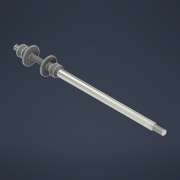
# Autodesk Inventor part: tłoczysko
Saved by Autodesk Inventor 2022 (Build 260153000, 153)
## iProperties
Created: 2023-04-12
Part Number: tłoczysko
Material: Ogólny
Document SubType Name: Modeling
Designer: jacek
Density: 1 g/cm^3
Appearance: Gładki — czarny
Author: jacek
Autodesk Inventor part; units mm, degrees
ref_plane "YZ Plane" through (0, 0, 0) normal (1, 0, 0) x (0, 1, 0)
ref_plane "XY Plane" through (0, 0, 0) normal (0, 0, 1) x (1, 0, 0)
sketch "Szkic1" plane through (0, 0, 0) normal (1, 0, 0) x (0, 1, 0)
  circle A0 centre (0, 0) radius 7
  dimension "d0" = 14
  constraints: 1 centre point, 1 coincident
  measures "d0" diameter of A0
extrude "Wyciągnięcie proste1" add sketch "Szkic1" along normal blind 100
sketch "Szkic2" plane through (100, 0, 0) normal (1, 0, 0) x (0, 0, -1)
  circle A0 centre (0, 0) radius 25.5
  dimension "d3" = 51
  constraints: 1 centre point, 1 coincident
  measures "d3" diameter of A0
extrude "Wyciągnięcie proste2" add sketch "Szkic2" against normal blind 3
ref_plane "Płaszczyzna konstrukcyjna1" through (43, 0, 0) normal (-1, 0, 0) x (0, 0, 1)
sketch "Szkic3" plane through (43, 0, 0) normal (-1, 0, 0) x (0, 0, 1)
  circle A0 centre (0, 0) radius 25.5
  constraints: 1 centre point, 1 coincident
extrude "Wyciągnięcie proste3" add sketch "Szkic3" along normal blind 3
sketch "Szkic4" plane through (40, 0, 0) normal (-1, 0, 0) x (0, 0, 1)
  circle A0 centre (0, 0) radius 10
  dimension "d9" = 20
  constraints: 1 centre point, 1 coincident
  measures "d9" diameter of A0
extrude "Wyciągnięcie proste4" add sketch "Szkic4" along normal blind 9
sketch "Szkic5" plane through (31, 0, 0) normal (-1, 0, 0) x (0, 0, 1)
  circle A0 centre (0, 0) radius 13.5
  dimension "d12" = 27
  constraints: 1 centre point, 1 coincident
  measures "d12" diameter of A0
extrude "Wyciągnięcie proste5" add sketch "Szkic5" along normal blind 11
fillet "Zaokrąglenie1" radius 8 1 edges at (31, 0, -13.5)
ref_plane "Płaszczyzna konstrukcyjna2" through (10, 0, 0) normal (-1, 0, 0) x (0, 0, 1)
sketch "Szkic6" plane through (10, 0, 0) normal (-1, 0, 0) x (0, 0, 1)
  circle A0 centre (0, 0) radius 14.5
  dimension "d19" = 29
  constraints: 1 centre point, 1 coincident
  measures "d19" diameter of A0
extrude "Wyciągnięcie proste6" add sketch "Szkic6" against normal blind 1
sketch "Szkic7" plane through (11, 0, 0) normal (1, 0, 0) x (0, 0, -1)
  circle A0 centre (0, 0) radius 15
  dimension "d22" = 30
  constraints: 1 centre point, 1 coincident
  measures "d22" diameter of A0
extrude "Wyciągnięcie proste7" add sketch "Szkic7" along normal blind 1
sketch "Szkic8" plane through (12, 0, 0) normal (1, 0, 0) x (0, 0, -1)
  circle A0 centre (0, 0) radius 7 projected
  circle A1 centre (0, 0) radius 15.75
  circle A2 centre (0, 0) radius 13.5 projected
  circle A3 centre (0, 0) radius 14.5
  dimension "d25" = 31.5
  constraints: 2 centre point, 2 coincident
  measures "d25" diameter of A1
extrude "Wyciągnięcie proste8" add sketch "Szkic8" along normal blind 13 contours A1
extrude "Wyciągnięcie proste9" add sketch "Szkic8" along normal blind 7.75 contours A0 | A2 | A3
sketch "Szkic9" plane through (100, 0, 0) normal (1, 0, 0) x (0, 0, -1)
  circle A0 centre (0, 0) radius 7
  circle A1 centre (0, 0) radius 10
  dimension "d30" = 14
  dimension "d33" = 20
  constraints: 2 centre point, 2 coincident
  measures "d30" diameter of A0
  measures "d33" diameter of A1
extrude "Wyciągnięcie proste10" add sketch "Szkic9" along normal blind 23 contours A0
extrude "Wyciągnięcie proste11" add sketch "Szkic9" along normal blind 9
sketch "Szkic10" plane through (109, 0, 0) normal (1, 0, 0) x (0, 0, -1)
  circle A0 centre (0, 0) radius 25.5 projected
  circle A1 centre (0, 0) radius 13.5
  dimension "d36" = 27
  constraints: 1 centre point, 1 coincident
  measures "d36" diameter of A1
extrude "Wyciągnięcie proste12" add sketch "Szkic10" along normal blind 11 contours A1
fillet "Zaokrąglenie2" radius 8 1 edges at (109, 0, 13.5)
ref_plane "Płaszczyzna konstrukcyjna3" through (115.5, 0, 0) normal (1, 0, 0) x (0, 0, -1)
sketch "Szkic11" plane through (115.5, 0, 0) normal (1, 0, 0) x (0, 0, -1)
  circle A0 centre (0, 0) radius 15.75
  circle A1 centre (0, 0) radius 14.5
  dimension "d41" = 31.5
  dimension "d42" = 29
  constraints: 2 centre point, 2 coincident
  measures "d41" diameter of A0
  measures "d42" diameter of A1
extrude "Wyciągnięcie proste13" add sketch "Szkic11" along normal blind 13
sketch "Szkic12" plane through (123, 0, 0) normal (1, 0, 0) x (0, 0, -1)
  circle A0 centre (0, 0) radius 10
  dimension "d45" = 20
  constraints: 1 centre point, 1 coincident
  measures "d45" diameter of A0
extrude "Wyciągnięcie proste14" add sketch "Szkic12" along normal blind 350
ref_plane "Płaszczyzna konstrukcyjna4" through (128.5, 0, 0) normal (1, 0, 0) x (0, 0, -1)
sketch "Szkic13" plane through (128.5, 0, 0) normal (1, 0, 0) x (0, 0, -1)
  circle A0 centre (0, 0) radius 15.75
  constraints: 1 centre point, 1 coincident
extrude "Wyciągnięcie proste15" add sketch "Szkic13" along normal blind 8
fillet "Zaokrąglenie3" radius 8 1 edges at (136.5, 0, 15.75)
sketch "Szkic14" plane through (473, 0, 0) normal (1, 0, 0) x (0, 0, -1)
  circle A0 centre (0, 0) radius 7.5
  circle A1 centre (0, 0) radius 18.8953
  dimension "d52" = 15
  constraints: 2 centre point, 2 coincident
  measures "d52" diameter of A0
extrude "Wyciągnięcie proste16" cut sketch "Szkic14" against normal blind 35
thread "Gwint2" size "M15x1.5" class "6g" standard "ANSI Metric M Profile" length 33
chamfer "Faza1" distance 2 angle 45 2 edges at (473, 0, 7.5) (438, 0, 10)
ref_plane "Płaszczyzna konstrukcyjna5" through (123, 10, 0) normal (0, 1, 0) x (-1, 0, 0)
sketch "Szkic15" plane through (123, 10, 0) normal (0, 1, 0) x (-1, 0, 0)
  line L0 (-290.266, 8.5) -> (-315.266, 8.5)
  line L1 (-315.266, 8.5) -> (-315.266, -8.5)
  line L2 (-315.266, -8.5) -> (-290.266, -8.5)
  line L3 (-290.266, -8.5) -> (-290.266, 8.5)
  line L4 (-290.266, 8.5) -> (-315.266, -8.5) construction
  line L5 (-315.266, 8.5) -> (-290.266, -8.5) construction
  line L6 (-317.1784, 11.3555) -> (-288.3535, 11.3555)
  line L7 (-288.3535, 11.3555) -> (-288.3535, -11.3555)
  line L8 (-288.3535, -11.3555) -> (-317.1784, -11.3555)
  line L9 (-317.1784, -11.3555) -> (-317.1784, 11.3555)
  line L10 (-317.1784, 11.3555) -> (-288.3535, -11.3555) construction
  line L11 (-288.3535, 11.3555) -> (-317.1784, -11.3555) construction
  line L12 (-290.266, -8.5) -> (-288.3535, -11.3555)
  line L13 (-290.266, 8.5) -> (-288.3535, 11.3555)
  line L14 (-315.266, -8.5) -> (-317.1784, -8.5)
  line L15 (-315.266, 8.5) -> (-317.1784, 8.5)
  point P0 (123, 0)
  point P1 (-302.766, 0)
  dimension "d60" = 25
  dimension "d61" = 17
  constraints: 32 end point, 4 midpoint, 4 parallel, 4 perpendicular, 2 horizontal, 2 point on line
  measures "d60" distance of L2.end L1.end
  measures "d61" distance of L1.end L0.end
extrude "Wyciągnięcie proste17" cut sketch "Szkic15" against normal blind 35 contours L0 L15 L9 L6 L13 | L12 L8 L9 L14 L2
sketch "Szkic16" plane through (0, 0, 0) normal (-1, 0, 0) x (0, 0, 1)
  circle A0 centre (0, 0) radius 7 projected
extrude "Wyciągnięcie proste18" add sketch "Szkic16" along normal blind 8
thread "Gwint3" size "M14x2" class "6g" standard "ANSI Metric M Profile" length 33
chamfer "Faza2" distance 2 angle 45 1 edges at (-8, 0, -7)
